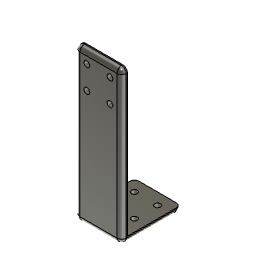
_acrylic lower bracket.b6740a63-519d-45cc-87e6-a969d2d498be (Autodesk Fusion 360 design; units mm, degrees)
Autodesk Fusion 360 part; units mm, degrees
note: some values were not read from the file. Set by a fixed rule: which sketch regions a step uses.
sketch "Sketch1" plane through (0, 0, 0) normal (0, 0, 1) x (1, 0, 0)
  line L0 (0, 0) -> (40, 0)
  line L1 (40, 0) -> (40, 51)
  line L2 (40, 51) -> (0, 51)
  line L3 (0, 51) -> (0, 0)
  dimension "d1" = 40
  dimension "d2" = 51
  constraint horizontal L0
  constraint vertical L1
  constraint horizontal L2
  constraint vertical L3
  constraint coincident L0.start L3.end
  measures "d1" distance of L0.start L0.end
  measures "d2" distance of L0.start L2.end
extrude "Extrude1" add sketch "Sketch1" along normal blind 5
sketch "Sketch2" plane through (0, 0, 5) normal (0, 0, 1) x (-1, 0, 0)
  line L0 (0, -51) -> (0, 0)
  line L1 (0, 0) -> (-40, 0)
  line L2 (-40, 0) -> (-40, -51)
  line L3 (-40, -51) -> (0, -51)
  line L4 (0, 0) -> (-40, 0)
  line L5 (-40, 0) -> (-40, -5)
  line L6 (-40, -5) -> (0, -5)
  line L7 (0, -5) -> (0, 0)
  dimension "d5" = 40
  dimension "d6" = 5
  constraint horizontal L4
  constraint vertical L5
  constraint horizontal L6
  constraint vertical L7
  constraint coincident L0.end L1.start
  measures "d5" distance of L0.end L1.end
  measures "d6" distance of L0.end L6.end
extrude "Extrude2" add sketch "Sketch2" along normal blind 126 contours L0 L1 L2 L4 L5 L6 L7
sketch "Sketch3" plane through (0, 0, 0) normal (0, -1, 0) x (1, 0, 0)
  line L0 (0, 0) -> (40, 0)
  line L1 (40, 0) -> (40, 131)
  line L2 (40, 131) -> (0, 131)
  line L3 (0, 131) -> (0, 0)
  line L4 (0, 131) -> (10, 131)
  line L5 (10, 131) -> (10, 121)
  line L6 (10, 121) -> (0, 121)
  line L7 (0, 121) -> (0, 131)
  circle A0 centre (10, 121) radius 2.5
  line L8 (10, 121) -> (30, 121)
  line L9 (30, 121) -> (30, 101)
  line L10 (30, 101) -> (10, 101)
  line L11 (10, 101) -> (10, 121)
  circle A1 centre (30, 121) radius 2.5
  circle A2 centre (10, 101) radius 2.5
  circle A3 centre (30, 101) radius 2.5
  dimension "d9" = 10
  dimension "d10" = 10
  dimension "d11" = 5
  dimension "d12" = 20
  dimension "d13" = 20
  dimension "d14" = 5
  dimension "d15" = 5
  dimension "d16" = 5
  constraint horizontal L4
  constraint vertical L5
  constraint horizontal L6
  constraint vertical L7
  constraint coincident L2.end L3.start
  constraint coincident L5.end L6.start
  constraint horizontal L8
  constraint vertical L9
  constraint horizontal L10
  constraint vertical L11
  constraint coincident L8.end L9.start
  constraint coincident L10.end L11.start
  constraint coincident L9.end L10.start
  measures "d9" distance of L2.end L4.end
  measures "d10" distance of L2.end L6.end
  measures "d11" diameter of A0
  measures "d12" distance of L5.end L8.end
  measures "d13" distance of L5.end L10.end
  measures "d14" diameter of A1
  measures "d15" diameter of A2
  measures "d16" diameter of A3
extrude "Extrude3" cut sketch "Sketch3" against normal blind 5 contours L5 L6 A0 | L6 A0 L11 | L5 A0 L8 | A0 L8 L11 | L10 L11 A2 | L10 L11 A2 | L8 L9 A1 | L8 L9 A1 | L9 L10 A3 | L9 L10 A3
sketch "Sketch4" plane through (0, 0, 5) normal (0, 0, 1) x (-1, 0, 0)
  line L0 (0, -5) -> (-40, -5)
  line L1 (-40, -5) -> (-40, -51)
  line L2 (-40, -51) -> (0, -51)
  line L3 (0, -51) -> (0, -5)
  line L4 (0, -51) -> (-10, -51)
  line L5 (-10, -51) -> (-10, -41)
  line L6 (-10, -41) -> (0, -41)
  line L7 (0, -41) -> (0, -51)
  line L8 (-10, -41) -> (-30, -41)
  line L9 (-30, -41) -> (-30, -21)
  line L10 (-30, -21) -> (-10, -21)
  line L11 (-10, -21) -> (-10, -41)
  circle A0 centre (-10, -41) radius 2.5
  circle A1 centre (-30, -41) radius 2.5
  circle A2 centre (-10, -21) radius 2.5
  circle A3 centre (-30, -21) radius 2.5
  dimension "d19" = 10
  dimension "d20" = 10
  dimension "d21" = 20
  dimension "d22" = 20
  dimension "d23" = 5
  dimension "d24" = 5
  dimension "d25" = 5
  dimension "d26" = 5
  constraint horizontal L4
  constraint vertical L5
  constraint horizontal L6
  constraint vertical L7
  constraint coincident L2.end L3.start
  constraint horizontal L8
  constraint vertical L9
  constraint horizontal L10
  constraint vertical L11
  constraint coincident L5.end L6.start
  constraint coincident L8.end L9.start
  constraint coincident L10.end L11.start
  constraint coincident L9.end L10.start
  measures "d19" distance of L2.end L4.end
  measures "d20" distance of L2.end L6.end
  measures "d21" distance of L5.end L8.end
  measures "d22" distance of L5.end L10.end
  measures "d23" diameter of A0
  measures "d24" diameter of A1
  measures "d25" diameter of A2
  measures "d26" diameter of A3
extrude "Extrude4" cut sketch "Sketch4" against normal blind 5 contours L5 L6 A0 | L6 L11 A0 | L5 L8 A0 | L8 L11 A0 | L10 L11 A2 | L10 L11 A2 | L8 L9 A1 | L8 L9 A1 | L9 L10 A3 | L9 L10 A3
fillet "Fillet1" radius 4 11 edges at (40, 25.5, 0) (20, 0, 0) (20, 51, 0) (40, 51, 2.5) (0, 51, 2.5) (0, 25.5, 0) (40, 0, 65.5) (40, 2.5, 131) (0, 0, 65.5) (0, 2.5, 131) (20, 0, 131)
